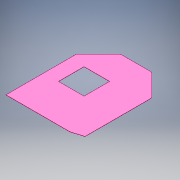
# Autodesk Inventor part: side plate
Saved by Autodesk Inventor 2018 (Build 220112000, 112)
## iProperties
Created: 2018-06-19
Part Number: side plate
Material: Steel
Document SubType Name: Sheet Metal
Designer: P446509
Density: 7.85 g/cm^3
Appearance: Pink
Sheet Metal Rule: Default
Author: P446509
Autodesk Inventor part; units mm, degrees
ref_plane "YZ Plane" through (0, 0, 0) normal (1, 0, 0) x (0, 1, 0)
ref_plane "XZ Plane" through (0, 0, 0) normal (0, 1, 0) x (-1, 0, 0)
ref_plane "XY Plane" through (0, 0, 0) normal (0, 0, 1) x (1, 0, 0)
sketch "Sketch1" plane through (0, 0, 0) normal (0, 0, 1) x (1, 0, 0)
  line L0 (-314, 325.9188) -> (-204, 325.9188)
  line L1 (-204, 325.9188) -> (-204, 545.9188)
  line L2 (-204, 545.9188) -> (-424, 545.9188)
  line L3 (-424, 545.9188) -> (-424, 325.9188)
  line L4 (-424, 325.9188) -> (-314, 325.9188)
  line L5 (0, 0) -> (100, 30)
  line L6 (0, 0) -> (272.914, 0) construction
  line L7 (100, 30) -> (100, 605)
  line L8 (0, 0) -> (-550, 0)
  line L9 (-550, 0) -> (-550, 605)
  line L10 (100, 605) -> (-90.9188, 795.9188)
  line L11 (100, 605) -> (370, 605) construction
  line L12 (-90.9188, 795.9188) -> (-359.0812, 795.9188)
  line L13 (-550, 605) -> (-359.0812, 795.9188)
  line L14 (-550, 605) -> (-280, 605) construction
  dimension "d10" = 110
  dimension "d11" = 220
  dimension "d12" = 220
  dimension "d21" = 100
  dimension "d24" = 550
  dimension "d25" = 126
  dimension "d29" = 30
  dimension "d30" = 270
  dimension "d31" = 135
  dimension "d32" = 270
  dimension "d33" = 45
  dimension "d34" = 605
  dimension "d35" = 250
  constraints: 30 end point, 6 horizontal, 3 perpendicular, 3 vertical, 2 equal length
  measures "d10" distance of L0.start L0.end
  measures "d11" distance of L0.end L1.end
  measures "d12" distance of L1.end L2.end
  measures "d21" distance from line of L5.start L7
  measures "d24" distance of L5.start L8.end
  measures "d25" distance between parallel lines of L9 L3
  measures "d29" distance from line of L8 L5.end
  measures "d30" distance of L7.end L10.end
  measures "d31" angle of L11 L10
  measures "d32" distance of L9.end L12.end
  measures "d33" angle of L14 L13
  measures "d34" distance of L9.end L8.end
  measures "d35" distance between parallel lines of L12 L2
extrude "Extrusion1" add sketch "Sketch1" along normal blind 1.6
fillet "Fillet2" radius 30 2 edges at (100, 605, 0.8) (-90.9188, 795.9188, 0.8)
equation "\"BendRadius\" = Thickness"
equation "\"BendReliefWidth\" = Thickness"
equation "\"BendReliefDepth\" = 0.5 * Thickness"
equation "\"CornerReliefSize\" = 4 * Thickness"
equation "\"MinimumRemnant\" = 2 * Thickness"
equation "\"TransitionRadius\" = BendRadius"
equation "\"JacobiRadiusSize\" = Thickness"
equation "\"GapSize\" = Thickness"
equation "\"Thickness\" = 0.5"
body "Solid1"
